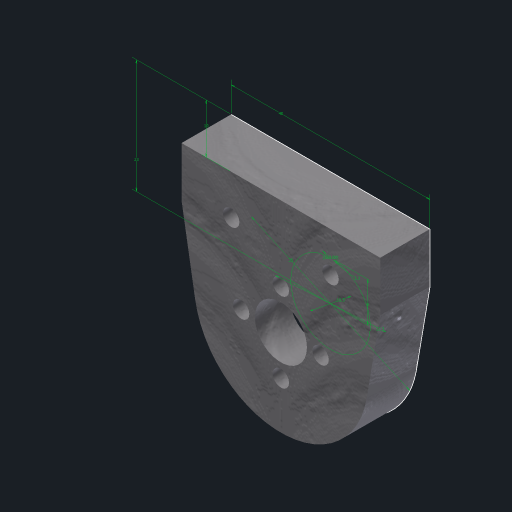
# Autodesk Inventor part: PARA_TUERCA
Saved by Autodesk Inventor 2024.3 (Build 283343000, 343)
## iProperties
Created: 2024-08-24
Part Number: PARA_TUERCA
Material: Steel, Mild, Welded
Document SubType Name: Modeling
Designer: Niler
Density: 7.85 g/cm^3
Appearance: Weld - Steel Mild
Author: Niler
Autodesk Inventor part; units mm, degrees
ref_plane "YZ Plane" through (0, 0, 0) normal (1, 0, 0) x (0, 1, 0)
ref_plane "XZ Plane" through (0, 0, 0) normal (0, 1, 0) x (-1, 0, 0)
ref_plane "XY Plane" through (0, 0, 0) normal (0, 0, 1) x (1, 0, 0)
sketch "Sketch1" plane through (0, 0, 0) normal (0, 0, 1) x (1, 0, 0)
  line L0 (-20, -5) -> (20, -5)
  line L1 (20, -5) -> (20, 5)
  line L2 (20, 5) -> (-20, 5)
  line L3 (-20, 5) -> (-20, -5)
  line L4 (-20, -5) -> (20, 5) construction
  line L5 (20, -5) -> (-20, 5) construction
  circle A0 centre (0, -18) radius 11.15
  circle A1 centre (0, -18) radius 5.25
  circle A2 centre (0, -18) radius 17.5
  line L6 (-20, -5) -> (-17.2455, -20.9738)
  line L7 (20, -5) -> (17.2455, -20.9738)
  circle A3 centre (0, -10) radius 1.65
  circle A4 centre (-8, -18) radius 1.65
  circle A5 centre (0, -26) radius 1.65
  circle A6 centre (8, -18) radius 1.65
  point P0 (0, 0)
  dimension "d0" = 22.3
  dimension "d1" = 10.5
  dimension "d2" = 35
  dimension "d3" = 3.3
  dimension "d4" = 8
  dimension "d7" = 360
  dimension "d14" = 40
  dimension "d16" = 23
  dimension "d17" = 10
  constraints: 16 end point, 7 centre point, 2 coincident, 2 midpoint, 2 parallel, 2 point on circle, 2 tangent, 2 vertical alignment, 1 horizontal, 1 perpendicular, 9 other
  measures "d0" diameter of A0
  measures "d1" diameter of A1
  measures "d2" diameter of A2
  measures "d3" diameter of A3
  measures "d4" distance of A0.centre A3.centre
  measures "d14" distance of L1.end L2.end
  measures "d16" distance from line of A0.centre L2
  measures "d17" distance of L2.end L0.start
extrude "Extrusion1" add sketch "Sketch1" along normal blind 10 contours L3 L2 L1 L0 A2 | L0 A2 L6 | A2 L0 | L0 A2 | L0 L7 A2 | A0
extrude "Extrusion2" cut sketch "Sketch1" along normal blind 3 contours A0
sketch "Sketch2" plane through (0, 0, 10) normal (0, 0, 1) x (1, 0, 0)
  line L0 (20, 5) -> (-20, 5) projected
  line L1 (-20, 5) -> (-20, -5) projected
  line L2 (-20, -5) -> (-17.2455, -20.9738) projected
  arc A0 (-17.2455, -20.9738) -> (17.2455, -20.9738) centre (0, -18) ccw projected
  line L3 (17.2455, -20.9738) -> (20, -5) projected
  line L4 (20, -5) -> (20, 5) projected
  circle A1 centre (0, -18) radius 5.25 projected
  circle A2 centre (0, -10) radius 1.65 projected
  circle A3 centre (-8, -18) radius 1.65 projected
  circle A4 centre (0, -26) radius 1.65 projected
  circle A5 centre (8, -18) radius 1.65 projected
  circle A6 centre (-10, -3) radius 1.65
  circle A7 centre (10, -3) radius 1.65
  line L5 (-10, -3) -> (10, -3)
  point P0 (0, 0)
  point P1 (0, -3)
  dimension "d18" = 3.3
  dimension "d19" = 3.3
  dimension "d20" = 8
  dimension "d21" = 20
  constraints: 2 centre point, 2 end point, 1 horizontal, 1 horizontal alignment, 1 midpoint, 1 vertical alignment
  measures "d18" diameter of A6
  measures "d19" diameter of A7
  measures "d20" distance between parallel lines of L0 L5
  measures "d21" distance of L5.start L5.end
extrude "Extrusion3" cut sketch "Sketch2" against normal through all contours A6 | A7
body "Solid1"
